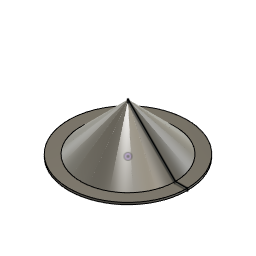
electrode puck v28 (Autodesk Fusion 360 archive; units mm, degrees)
design "electrode"
Autodesk Fusion 360 part; units mm, degrees
sketch "Sketch1" plane through (0, 0, 0) normal (0, 0, 1) x (1, 0, 0)
  line L0 (2.4, 0.1) -> (0, 2.5)
  line L1 (0, 2.5) -> (0, 2.3586)
  line L2 (0, 2.3586) -> (2.3586, 0)
  line L3 (2.3586, 0) -> (3, 0)
  line L4 (3, 0) -> (3, 0.1)
  line L5 (3, 0.1) -> (2.4, 0.1)
  dimension "d1" = 0.1
  dimension "d2" = 0.1
  dimension "d3" = 2.4
  dimension "d4" = 45
  dimension "d5" = 3
  constraint vertical L1
  constraint parallel L0 L2
  constraint horizontal L3
  constraint perpendicular L3 L4
  constraint perpendicular L4 L5
  constraint coincident origin L1
  constraint coincident origin L3
  measures "d1" distance of L3 L5
  measures "d2" distance of L0 L2
  measures "d3" horizontal distance of origin L0.start
  measures "d4" angle of L2 L3
  measures "d5" distance of origin L4
revolve "Revolve1" add sketch "Sketch1" angle 360 about axis through (0, 1.75, 0) along (0, 1, 0)
hole "Hole1" at (0, 0, 0) direction (0, 1, 0) diameter 0.05 end through all
